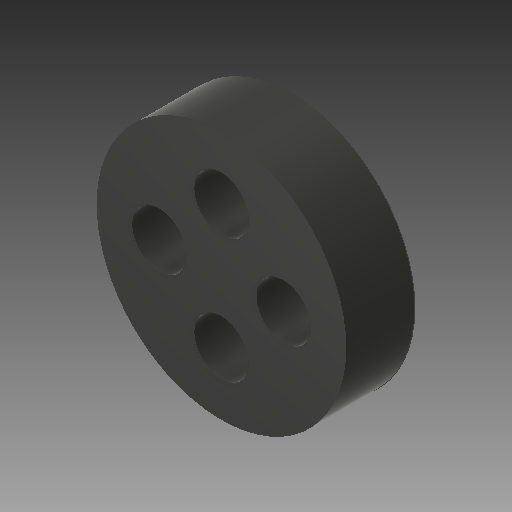
# Autodesk Inventor part: アーム中間節カム1
Saved by Autodesk Inventor 2020 (Build 240168000, 168)
## iProperties
Created: 2018-11-21
Part Number: アーム中間節カム1
Material: アセタール樹脂、黒
Document SubType Name: Modeling
Designer: 雪村
Density: 1.425 g/cm^3
Appearance: 滑らか - 黒
Mass: 1.45495 g
Surface Area: 9.42478 cm^2
Volume: 1.02102 cm^3
Description: ジュラコン 5t
Author: 雪村
Autodesk Inventor part; units mm, degrees
ref_plane "YZ Plane" through (0, 0, 0) normal (1, 0, 0) x (0, 1, 0)
ref_plane "XZ Plane" through (0, 0, 0) normal (0, 1, 0) x (-1, 0, 0)
ref_plane "XY Plane" through (0, 0, 0) normal (0, 0, 1) x (1, 0, 0)
sketch "スケッチ1" plane through (0, 0, 0) normal (0, 0, 1) x (1, 0, 0)
  circle A0 centre (0, 0) radius 9
  circle A1 centre (-4.5, 0) radius 4.5 construction
  circle A2 centre (4.5, 0) radius 4.5 construction
  circle A3 centre (-4.5, 0) radius 2
  circle A4 centre (4.5, 0) radius 2
  line L0 (4.5, 0) -> (0, -4.5) construction
  line L1 (0, -4.5) -> (-4.5, 0) construction
  line L2 (-4.5, 0) -> (0, 4.5) construction
  line L3 (0, 4.5) -> (4.5, 0) construction
  circle A5 centre (0, 4.5) radius 2
  circle A6 centre (0, -4.5) radius 2
  dimension "d1" = 9
  dimension "d0" = 18
  dimension "d2" = 9
  dimension "d3" = 4
  dimension "d4" = 4
  dimension "d14" = 4
  dimension "d15" = 4
  constraints: 8 end point, 6 centre point, 6 coincident, 3 horizontal alignment, 12 other
  measures "d0" diameter of A0
  measures "d2" diameter of A2
  measures "d3" diameter of A3
  measures "d4" diameter of A4
  measures "d14" diameter of A5
  measures "d15" diameter of A6
extrude "押し出し1" add sketch "スケッチ1" along normal blind 5
